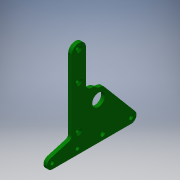
# Autodesk Inventor part: support plate 2
Saved by Autodesk Inventor 2017 SP1 (Build 210196100, 196)
## iProperties
Created: 2018-01-20
Part Number: support plate 2
Material: Aluminum 6061
Document SubType Name: Modeling
Designer: Ben
Density: 2.7 g/cm^3
Appearance: Dark Green
Mass: 193.553 g
Surface Area: 279.348 cm^2
Volume: 71.6862 cm^3
Author: Ben
Autodesk Inventor part; units mm, degrees
ref_plane "YZ Plane" through (0, 0, 0) normal (1, 0, 0) x (0, 1, 0)
ref_plane "XZ Plane" through (0, 0, 0) normal (0, 1, 0) x (-1, 0, 0)
ref_plane "XY Plane" through (0, 0, 0) normal (0, 0, 1) x (1, 0, 0)
sketch "Sketch1" plane through (0, 0, 0) normal (1, 0, 0) x (0, 1, 0)
  circle A0 centre (0, 0) radius 2.667
  circle A1 centre (76.2, 0) radius 2.667
  circle A2 centre (127, 0) radius 2.667
  line L0 (127, 0) -> (0, 0) construction
  line L1 (0, 12.7) -> (123.825, 12.7)
  line L2 (123.825, -12.7) -> (66.04, -12.7)
  line L3 (-12.7, -95.2899) -> (-12.7, 0) construction
  line L4 (-12.7, 0) -> (0, 0) construction
  line L5 (136.525, 0) -> (127, 0) construction
  arc A3 (123.825, -12.7) -> (123.825, 12.7) centre (123.825, 0) ccw
  arc A4 (-34.0868, -92.837) -> (-18.4185, -100.1161) centre (-24.5618, -92.837) ccw
  arc A5 (66.04, -12.7) -> (56.515, -22.225) centre (66.04, -22.225) ccw
  circle A6 centre (31.75, -34.925) radius 11.1125
  circle A7 centre (31.75, -34.925) radius 12.7 construction
  line L6 (31.75, -22.225) -> (149.0837, -22.225) construction
  line L7 (56.515, 0) -> (56.515, -22.225) construction
  circle A8 centre (-24.5618, 46.863) radius 3.3528
  circle A9 centre (-24.2985, 2.0822) radius 3.3528
  circle A10 centre (-24.5618, -42.7) radius 4.064
  circle A11 centre (-24.5618, -92.837) radius 3.3528
  arc A12 (-15.4112, 49.5073) -> (-34.0868, 46.863) centre (-24.5618, 46.863) ccw
  line L8 (-34.0868, 46.863) -> (-34.0868, -92.837)
  line L9 (-24.5618, 46.863) -> (-24.5618, -92.837) construction
  arc A13 (-6.1004, 17.2871) -> (0, 12.7) centre (0, 19.05) ccw
  line L10 (-6.1004, 17.2871) -> (-15.4112, 49.5073)
  line L11 (46.7971, -45.0762) -> (-18.4185, -100.1161)
  line L12 (43.0128, -48.27) -> (38.9172, -43.4173) construction
  arc A14 (53.2765, -30.1625) -> (56.515, -22.225) centre (45.1684, -22.225) ccw
  arc A15 (53.2765, -30.1625) -> (50.038, -38.1) centre (61.3846, -38.1) ccw
  arc A16 (46.7971, -45.0762) -> (50.038, -38.1) centre (40.9094, -38.1) ccw
  line L13 (50.038, -38.1) -> (50.038, -22.225) construction
  dimension "d33" = 22.225
  dimension "d34" = 25.4
  dimension "d0" = 5.334
  dimension "d1" = 127
  dimension "d3" = 12.7
  dimension "d13" = 25.4
  dimension "d14" = 9.525
  dimension "d20" = 9.525
  dimension "d35" = 44.45
  dimension "d37" = 76.2
  dimension "d38" = 69.215
  dimension "d39" = 22.225
  dimension "d40" = 9.525
  dimension "d42" = 11.5985
  dimension "d45" = 6.7056
  dimension "d46" = 11.8618
  dimension "d47" = 8.128
  dimension "d52" = 44.7808
  dimension "d53" = 44.7822
  dimension "d54" = 50.137
  dimension "d55" = 46.863
  dimension "d56" = 6.35
  dimension "d57" = 0
  dimension "d58" = 6.35
  dimension "d60" = 62.738
  dimension "d62" = 15.875
  constraints: 28 end point, 17 point on circle, 15 centre point, 13 tangent, 8 point on line, 7 equal radius, 4 coincident, 4 horizontal, 4 vertical, 3 perpendicular, 1 collinear, 1 vertical alignment, 5 other
  measures "d0" diameter of A0
  measures "d1" distance of L0.start L0.end
  measures "d3" distance from line of point (0, 0) L3
  measures "d13" distance between parallel lines of L1 L2
  measures "d14" distance of L5.start L0.start
  measures "d20" radius of A5
  measures "d35" distance from line of L3 point (31.75, -34.925)
  measures "d37" distance of point (0, 0) A1.centre
  measures "d38" distance between parallel lines of L3 L7
  measures "d39" distance between parallel lines of L0 L6
  measures "d40" radius of A12
  measures "d42" distance from line of A9.centre L3
  measures "d45" diameter of A8
  measures "d46" distance between parallel lines of L3 L9
  measures "d47" diameter of A10
  measures "d52" vertical distance of A9.centre A8.centre
  measures "d53" vertical distance of A10.centre A9.centre
  measures "d54" distance of A4.centre A10.centre
  measures "d55" distance from line of L4 A8.centre
  measures "d56" radius of A13
  measures "d57" horizontal distance of point (0, 0) L1.start
  measures "d58" distance of L12.start L12.end
  measures "d60" distance between parallel lines of L3 L13
  measures "d62" distance of L13.start L13.end
extrude "Extrusion1" add sketch "Sketch1" along normal mid plane 6.35
chamfer "Chamfer1" distance 3.175 angle 45 3 edges at (3.175, 124.333, 0) (3.175, 73.533, 0) (3.175, -2.667, 0)
body "Solid1"
